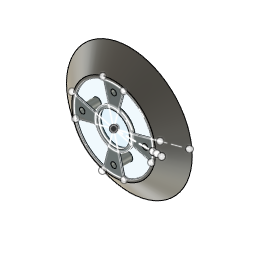
Shield (Autodesk Fusion 360 design; units mm, degrees)
Autodesk Fusion 360 part; units mm, degrees
sketch "Sketch1" plane through (0, 0, 0) normal (0, 0, 1) x (1, 0, 0)
  line L0 (0, 17) -> (0, -15) construction
  line L1 (0, 0) -> (40, 0)
  line L2 (0, 0) -> (0, 15)
  line L3 (0, 15) -> (60, 15)
  line L4 (40, 0) -> (60, 15)
  dimension "d1" = 40
  dimension "d2" = 15
  dimension "d3" = 60
  constraint vertical L0
  constraint coincident L1.start L2.start
  constraint perpendicular L0 L1
  constraint perpendicular L1 L2
  constraint perpendicular L0 L3
  measures "d1" distance of L1.start L1.end
  measures "d2" distance of L1.start L2.end
  measures "d3" distance of L2.end L3.end
revolve "Revolve1" add sketch "Sketch1" angle 360 about axis through (0, 17, 0) along (0, -1, 0)
shell "Shell1" thickness 1.2 removed faces 1 at (28.282, 15, -12.1475)
sketch "Sketch2" plane through (0, 1.2, 0) normal (0, 1, 0) x (-1, 0, 0)
  circle A0 centre (0, 0) radius 39.6
  circle A1 centre (0, 0) radius 30 construction
  line L0 (0, 37) -> (0, -35) construction
  line L1 (-35, 0) -> (37.2005, 0) construction
  circle A2 centre (0, 30) radius 2.6
  circle A3 centre (-30, 0) radius 2.6
  circle A4 centre (30, 0) radius 2.6
  circle A5 centre (0, -30) radius 2.6
  circle A6 centre (-30, 0) radius 4
  circle A7 centre (0, -30) radius 4
  circle A8 centre (30, 0) radius 4
  circle A9 centre (0, 30) radius 4
  dimension "d6" = 60
  dimension "d7" = 72
  dimension "d8" = 72.2005
  dimension "d9" = 5.2
  dimension "d10" = 5.2
  dimension "d11" = 5.2
  dimension "d12" = 5.2
  dimension "d13" = 8
  dimension "d14" = 8
  dimension "d15" = 8
  dimension "d16" = 8
  constraint coincident A0.centre A1.centre
  constraint vertical L0
  constraint horizontal L1
  constraint coincident L0 A2.centre
  constraint coincident A1 A2.centre
  constraint coincident L1 A3.centre
  constraint coincident A1 A3.centre
  constraint coincident L1 A4.centre
  constraint coincident A1 A4.centre
  constraint coincident L0 A5.centre
  constraint coincident A1 A5.centre
  constraint concentric A3 A6
  constraint concentric A5 A7
  constraint concentric A4 A8
  constraint concentric A2 A9
  measures "d6" diameter of A1
  measures "d7" distance of L0.start L0.end
  measures "d8" distance of L1.start L1.end
  measures "d9" diameter of A2
  measures "d10" diameter of A3
  measures "d11" diameter of A4
  measures "d12" diameter of A5
  measures "d13" diameter of A6
  measures "d14" diameter of A7
  measures "d15" diameter of A8
  measures "d16" diameter of A9
extrude "Extrude1" add sketch "Sketch2" along normal blind 13 contours A6 | A7 | A8 | A9
extrude "Extrude2" cut 4 faces at (0.8667, 1.2, 31.3552) (-30.7993, 1.2, -0.1292) (0.0929, 1.2, -30.6776) (30.6738, 1.2, -0.8449) along direction (0, -1, 0) blind 5
sketch "Sketch3" plane through (0, 1.2, 0) normal (0, 1, 0) x (-1, 0, 0)
  circle A0 centre (-30, 0) radius 4
  circle A1 centre (0, -30) radius 4
  circle A2 centre (0, 0) radius 39.6
  circle A3 centre (30, 0) radius 4
  circle A4 centre (0, 30) radius 4
  circle A5 centre (0, 0) radius 15.25
  dimension "d21" = 30.5
  constraint coincident A2.centre A5.centre
  measures "d21" diameter of A5
extrude "Extrude3" cut sketch "Sketch3" against normal blind 5 contours A5
sketch "Sketch4" plane through (0, 1.2, 0) normal (0, 1, 0) x (-1, 0, 0)
  line L0 (0, 0) -> (30, 30) construction
  circle A0 centre (0, 0) radius 20 construction
  circle A1 centre (14.1421, 14.1421) radius 2.6
  dimension "d24" = 42.4264
  dimension "d25" = 40
  dimension "d26" = 5.2
  constraint coincident L0.start A0.centre
  constraint coincident A0 A1.centre
  constraint coincident L0 A1.centre
  measures "d24" distance of L0.start L0.end
  measures "d25" diameter of A0
  measures "d26" diameter of A1
sketch "Sketch5" plane through (0, 0, 0) normal (0, 1, 0) x (1, 0, 0)
  circle A0 centre (0, 0) radius 37.5
  circle A1 centre (0, 0) radius 17.5
  line L0 (0, 0) -> (9.9905, 37.2852)
  line L1 (0, 0) -> (38.6005, 0) construction
  line L2 (0, 0) -> (-10.2701, -38.3286)
  line L3 (0, 0) -> (39.6807, 0) construction
  line L4 (0, 0) -> (-10.6714, 39.8261)
  line L5 (0, 0) -> (41.2311, 0) construction
  line L6 (0, 0) -> (9.7057, -36.2222)
  line L7 (0, 0) -> (37.5, 0) construction
  line L8 (0, 0) -> (72.4444, -19.4114) construction
  line L9 (0, 0) -> (-36.2222, 9.7057)
  line L10 (0, 0) -> (37.5, 0) construction
  line L11 (0, 0) -> (36.2222, 9.7057)
  line L12 (0, 0) -> (37.5, 0) construction
  line L13 (0, 0) -> (-39.8261, -10.6714)
  line L14 (0, 0) -> (41.2311, 0) construction
  line L15 (0, 0) -> (44.3411, -11.8812)
  line L16 (0, 0) -> (45.9235, 0) construction
  dimension "d29" = 75
  dimension "d30" = 35
  dimension "d31" = 75
  dimension "d32" = 105
  dimension "d33" = 105
  dimension "d34" = 75
  dimension "d35" = 75
  dimension "d36" = 165
  dimension "d37" = 15
  dimension "d38" = 165
  dimension "d39" = 15
  constraint coincident A0.centre A1.centre
  constraint horizontal L1
  constraint horizontal L3
  constraint horizontal L5
  constraint horizontal L7
  constraint horizontal L10
  constraint horizontal L12
  constraint horizontal L14
  constraint horizontal L16
  constraint parallel L8 L15
  measures "d29" diameter of A0
  measures "d30" diameter of A1
  measures "d31" angle of L0 L1
  measures "d32" angle of L2 L3
  measures "d33" angle of L4 L5
  measures "d34" angle of L6 L7
  measures "d35" distance of A0.centre L8.end
  measures "d36" angle of L9 L10
  measures "d37" angle of L11 L12
  measures "d38" angle of L13 L14
  measures "d39" angle of L15 L16
extrude "Extrude5" cut sketch "Sketch5" along normal blind 5 contours A0 A1 L0 L11 | A0 A1 L6 L15 | A0 A1 L4 L9 | A0 A1 L2 L13
sketch "Sketch6" plane through (0, 1.2, 0) normal (0, 1, 0) x (-1, 0, 0)
  circle A0 centre (0, 0) radius 17.5
  circle A1 centre (0, 0) radius 15.25
  dimension "d42" = 35
  dimension "d43" = 30.5
  constraint coincident A0.centre A1.centre
  measures "d42" diameter of A0
  measures "d43" diameter of A1
extrude "Extrude6" add sketch "Sketch6" along normal blind 2
fillet "Fillet1" radius 2 1 edges at (36.2222, 0.6, -9.7057)
fillet "Fillet1" radius 2 1 edges at (16.9037, 0.6, -4.5293)
fillet "Fillet1" radius 2 1 edges at (4.5293, 0.6, -16.9037)
fillet "Fillet1" radius 2 1 edges at (9.7057, 0.6, -36.2222)
fillet "Fillet2" radius 2 1 edges at (9.7057, 0.6, 36.2222)
fillet "Fillet3" radius 2 1 edges at (4.5293, 0.6, 16.9037)
fillet "Fillet4" radius 2 1 edges at (16.9037, 0.6, 4.5293)
fillet "Fillet5" radius 2 1 edges at (36.2222, 0.6, 9.7057)
fillet "Fillet6" radius 2 1 edges at (-4.5293, 0.6, 16.9037)
fillet "Fillet7" radius 2 1 edges at (-16.9037, 0.6, 4.5293)
fillet "Fillet8" radius 2 1 edges at (-9.7057, 0.6, 36.2222)
fillet "Fillet9" radius 2 1 edges at (-36.2222, 0.6, 9.7057)
fillet "Fillet10" radius 2 1 edges at (-9.7057, 0.6, -36.2222)
fillet "Fillet11" radius 2 1 edges at (-4.5293, 0.6, -16.9037)
fillet "Fillet12" radius 2 1 edges at (-16.9037, 0.6, -4.5293)
fillet "Fillet13" radius 2 1 edges at (-36.2222, 0.6, -9.7057)
